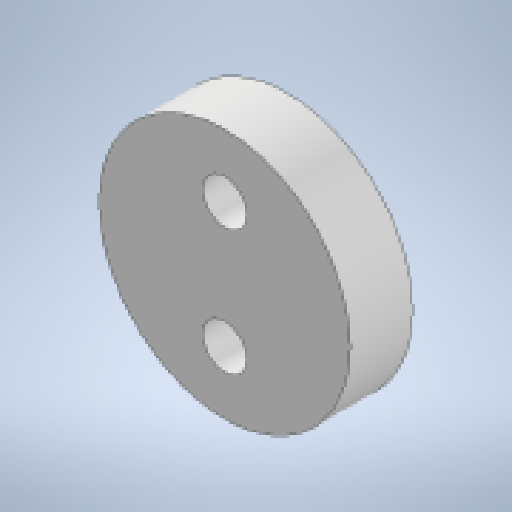
# Autodesk Inventor part: Motor Adapter
Saved by Autodesk Inventor 2023 (Build 270158000, 158)
## iProperties
Created: 2023-01-18
Part Number: Motor Adapter
Material: Generic
Document SubType Name: Modeling
Designer: caden
Density: 1 g/cm^3
Appearance: Default
Author: caden
Autodesk Inventor part; units mm, degrees
ref_plane "YZ Plane" through (0, 0, 0) normal (1, 0, 0) x (0, 1, 0)
ref_plane "XZ Plane" through (0, 0, 0) normal (0, 1, 0) x (-1, 0, 0)
ref_plane "XY Plane" through (0, 0, 0) normal (0, 0, 1) x (1, 0, 0)
sketch "Sketch2" plane through (0, 0, 0) normal (0, 0, 1) x (1, 0, 0)
  circle A0 centre (0, 0) radius 9.5
  dimension "d0" = 19
  constraints: 1 centre point, 1 coincident
  measures "d0" diameter of A0
extrude "Extrusion1" add sketch "Sketch2" along normal blind 11
sketch "Sketch5" plane through (0, 0, 11) normal (0, 0, 1) x (1, 0, 0)
  circle A0 centre (0, 0) radius 15
  dimension "d17" = 30
  constraints: 1 centre point, 1 coincident
  measures "d17" diameter of A0
extrude "Extrusion4" add sketch "Sketch5" against normal blind 5
sketch "Sketch3" plane through (0, 0, 11) normal (0, 0, 1) x (1, 0, 0)
  circle A0 centre (0, -4) radius 1.75
  circle A1 centre (0, 4) radius 1.75
  line L0 (0, -9.5) -> (0, 9.5) construction
  circle A2 centre (0, 0) radius 9.5 construction
  dimension "d3" = 3.5
  dimension "d4" = 3.5
  dimension "d5" = 8
  dimension "d6" = 4
  constraints: 2 centre point, 2 end point, 2 point on line, 1 coincident, 1 midpoint, 1 vertical, 1 vertical alignment, 1 other
  measures "d3" diameter of A0
  measures "d4" diameter of A1
  measures "d5" distance of A1.centre A0.centre
  measures "d6" distance of point (0, 0) A0.centre
extrude "Extrusion2" cut sketch "Sketch3" against normal through all
sketch "Sketch4" plane through (0, 0, 11) normal (0, 0, 1) x (1, 0, 0)
  circle A0 centre (-10, 0) radius 2.1
  circle A1 centre (10, 0) radius 2.1
  line L0 (10, 0) -> (-10, 0) construction
  point P0 (0, 0)
  point P1 (0, 0)
  dimension "d9" = 4.2
  dimension "d10" = 4.2
  dimension "d11" = 20
  constraints: 2 centre point, 2 end point, 1 coincident, 1 horizontal, 1 midpoint
  measures "d9" diameter of A0
  measures "d10" diameter of A1
  measures "d11" distance of L0.end L0.start
extrude "Extrusion3" cut sketch "Sketch4" against normal blind 5
chamfer "Chamfer1" distance 0.5 angle 45 2 edges at (7.9, 0, 11) (-12.1, 0, 11)
equation "\"d5\" = 2 * d6"
body "Solid1"
